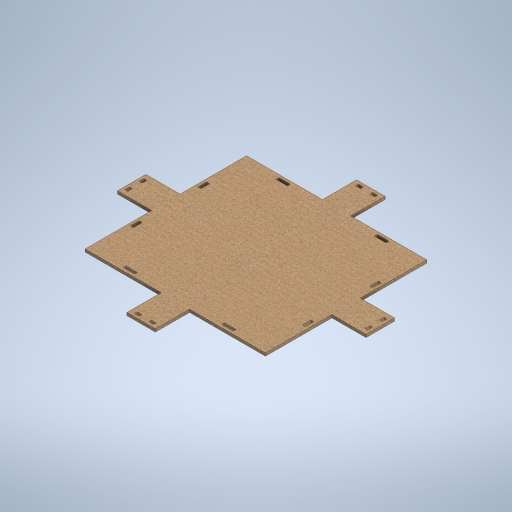
# Autodesk Inventor part: Base1
Saved by Autodesk Inventor 2024 (Build 280153000, 153)
## iProperties
Created: 2023-11-22
Part Number: Base1
Material: MDF Tablero de fibras de densidad media
Document SubType Name: Modeling
Designer: marco
Density: 0.8 g/cm^3
Appearance: Cartón - Ondulado
Author: marco
Autodesk Inventor part; units mm, degrees
ref_plane "YZ Plane" through (0, 0, 0) normal (1, 0, 0) x (0, 1, 0)
ref_plane "XZ Plane" through (0, 0, 0) normal (0, 1, 0) x (-1, 0, 0)
ref_plane "XY Plane" through (0, 0, 0) normal (0, 0, 1) x (1, 0, 0)
sketch "Boceto1" plane through (0, 0, 0) normal (0, 1, 0) x (-1, 0, 0)
  line L0 (-15, 118) -> (-15, 115)
  line L1 (-15, 121) -> (-15, 118)
  line L2 (-5, 115) -> (-10, 115)
  line L3 (-10, 115) -> (-10, 118)
  line L4 (-10, 118) -> (-5, 118)
  line L5 (-5, 118) -> (-5, 115)
  line L6 (10, 115) -> (5, 115)
  line L7 (5, 115) -> (5, 118)
  line L8 (5, 118) -> (10, 118)
  line L9 (10, 118) -> (10, 115)
  line L10 (-15, -85) -> (-15, -91)
  line L11 (-15, -121) -> (-15, -85)
  line L12 (-15, -121) -> (15, -121)
  line L13 (95, -15) -> (95, -85)
  line L14 (95, -85) -> (15, -85)
  line L15 (15, -85) -> (15, -121)
  line L16 (-15, 121) -> (-15, 85)
  line L17 (-15, 85) -> (-95, 85)
  line L18 (-95, 85) -> (-95, 15)
  line L19 (-95, 15) -> (-131, 15)
  line L20 (-131, 15) -> (-131, -15)
  line L21 (-131, -15) -> (-95, -15)
  line L22 (-95, -15) -> (-95, -85)
  line L23 (-95, -85) -> (-15, -85)
  line L24 (-10, -115) -> (-5, -115)
  line L25 (-5, -115) -> (-5, -118)
  line L26 (-5, -118) -> (-10, -118)
  line L27 (-10, -118) -> (-10, -115)
  line L28 (10, -115) -> (10, -118)
  line L29 (10, -118) -> (5, -118)
  line L30 (5, -118) -> (5, -115)
  line L31 (5, -115) -> (10, -115)
  line L32 (46, -82) -> (46, -79)
  line L33 (46, -79) -> (58, -79)
  line L34 (58, -79) -> (58, -82)
  line L35 (58, -82) -> (46, -82)
  line L36 (95, 15) -> (95, 21)
  line L37 (95, -15) -> (95, -21)
  line L38 (131, -15) -> (131, 15)
  line L39 (131, -15) -> (95, -15)
  line L40 (95, 15) -> (131, 15)
  line L41 (95, 15) -> (95, 85)
  line L42 (95, 85) -> (15, 85)
  line L43 (15, 85) -> (15, 121)
  line L44 (15, 121) -> (-15, 121)
  line L45 (125, 10) -> (125, 5)
  line L46 (125, 5) -> (128, 5)
  line L47 (128, 5) -> (128, 10)
  line L48 (128, 10) -> (125, 10)
  line L49 (128, -10) -> (125, -10)
  line L50 (125, -10) -> (125, -5)
  line L51 (125, -5) -> (128, -5)
  line L52 (128, -5) -> (128, -10)
  line L53 (92, -31) -> (92, -40)
  line L54 (92, -40) -> (89, -40)
  line L55 (89, -40) -> (89, -31)
  line L56 (89, -31) -> (92, -31)
  line L57 (92, 40) -> (92, 31)
  line L58 (92, 31) -> (89, 31)
  line L59 (89, 31) -> (89, 40)
  line L60 (89, 40) -> (92, 40)
  line L61 (46, 82) -> (46, 79)
  line L62 (46, 79) -> (58, 79)
  line L63 (58, 79) -> (58, 82)
  line L64 (58, 82) -> (46, 82)
  line L65 (-58, 82) -> (-58, 79)
  line L66 (-58, 79) -> (-46, 79)
  line L67 (-46, 79) -> (-46, 82)
  line L68 (-46, 82) -> (-58, 82)
  line L69 (-92, 31) -> (-92, 40)
  line L70 (-92, 40) -> (-89, 40)
  line L71 (-89, 40) -> (-89, 31)
  line L72 (-89, 31) -> (-92, 31)
  line L73 (-92, -31) -> (-92, -40)
  line L74 (-92, -40) -> (-89, -40)
  line L75 (-89, -40) -> (-89, -31)
  line L76 (-89, -31) -> (-92, -31)
  line L77 (-46, -82) -> (-46, -79)
  line L78 (-46, -79) -> (-58, -79)
  line L79 (-58, -79) -> (-58, -82)
  line L80 (-58, -82) -> (-46, -82)
  line L81 (-128, -5) -> (-128, -10)
  line L82 (-128, -10) -> (-125, -10)
  line L83 (-125, -10) -> (-125, -5)
  line L84 (-125, -5) -> (-128, -5)
  line L85 (-125, 10) -> (-125, 5)
  line L86 (-125, 5) -> (-128, 5)
  line L87 (-128, 5) -> (-128, 10)
  line L88 (-128, 10) -> (-125, 10)
  constraints: 178 end point
extrude "Extrusión1" add sketch "Boceto1" along normal blind 3
